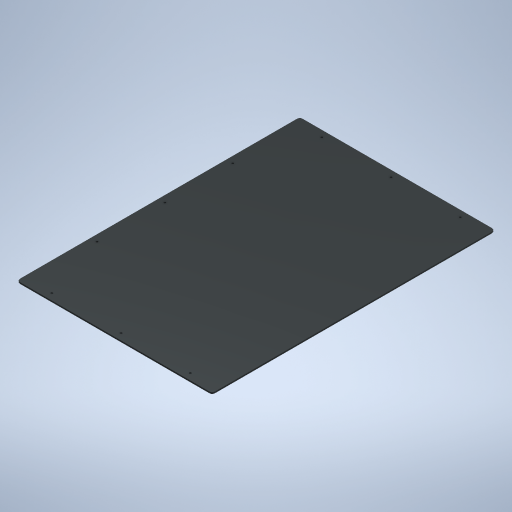
# Autodesk Inventor part: 1040x1000 esquina
Saved by Autodesk Inventor 2024.2 (Build 282272000, 272)
## iProperties
Created: 2025-10-02
Part Number: 1040x1000 esquina
Material: Hierro, fundido
Document SubType Name: Modeling
Designer: jd.castellanosq
Density: 7.15 g/cm^3
Appearance: Gris hierro
Author: jd.castellanosq
Autodesk Inventor part; units mm, degrees
ref_plane "YZ Plane" through (0, 0, 0) normal (1, 0, 0) x (0, 1, 0)
ref_plane "XZ Plane" through (0, 0, 0) normal (0, 1, 0) x (-1, 0, 0)
ref_plane "XY Plane" through (0, 0, 0) normal (0, 0, 1) x (1, 0, 0)
sketch "Boceto1" plane through (0, 0, 0) normal (0, 0, 1) x (1, 0, 0)
  line L0 (-345, 500) -> (345, 500)
  line L1 (345, 500) -> (345, -500)
  line L2 (345, -500) -> (-345, -500)
  line L3 (-345, -500) -> (-345, 500)
  circle A0 centre (-245, 477.5) radius 4
  circle A1 centre (245, 477.5) radius 4
  circle A2 centre (0, 477.5) radius 4
  circle A3 centre (245, 477.5) radius 4
  circle A4 centre (-245, -477.5) radius 4
  circle A5 centre (0, -477.5) radius 4
  circle A6 centre (245, -477.5) radius 4
  circle A7 centre (245, -477.5) radius 4
  circle A8 centre (-322.5, 240) radius 4
  circle A9 centre (-322.5, 0) radius 4
  circle A10 centre (-322.5, -240) radius 4
  point P0 (0, 0)
  point P1 (0, 500)
  point P2 (345, 0)
  point P3 (-345, 0)
  dimension "d0" = 690
  dimension "d4" = 1000
  dimension "d5" = 8
  dimension "d6" = 22.5
  dimension "d7" = 100
  dimension "d8" = 100
  dimension "d9" = 245
  dimension "d10" = 245
  dimension "d11" = 22.5
  dimension "d12" = 22.5
  dimension "d14" = 240
  dimension "d15" = 240
  constraints: 11 centre point, 10 equal radius, 8 end point, 7 horizontal alignment, 7 vertical alignment, 3 midpoint, 2 parallel, 1 coincident, 1 horizontal, 1 perpendicular
  measures "d0" distance of L0.start L0.end
  measures "d4" distance of L0.end L1.end
  measures "d5" diameter of A0
  measures "d6" distance from line of L0 A0.centre
  measures "d7" distance from line of A0.centre L3
  measures "d8" distance from line of L1 A1.centre
  measures "d9" distance of A2.centre A0.centre
  measures "d10" distance of A3.centre A2.centre
  measures "d11" distance from line of A4.centre L2
  measures "d12" distance from line of A9.centre L3
  measures "d14" distance of A9.centre A8.centre
  measures "d15" distance of A10.centre A9.centre
extrude "Extrusión1" add sketch "Boceto1" along normal blind 5
fillet "Empalme1" radius 10 4 edges at (345, 500, 2.5) (-345, 500, 2.5) (345, -500, 2.5) (-345, -500, 2.5)
equation "\"d8\" = d7"
equation "\"d10\" = d9"
equation "\"d11\" = d6"
equation "\"d12\" = d11"
equation "\"d15\" = d14"
